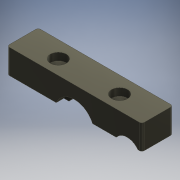
# Autodesk Inventor part: Retainer
Saved by Autodesk Inventor 2016 (Build 200138000, 138)
## iProperties
Created: 2016-11-19
Part Number: Retainer
Material: PC/ABS Plastic
Document SubType Name: Modeling
Designer: Scott
Density: 0.357273 g/cm^3
Appearance: Gunmetal
Author: Scott
## iProperties of the stored document Retainer_3DPrint.ipt
Created: 2017-03-26
Part Number: Retainer_3DPrint
Material: Generic
Document SubType Name: Modeling
Designer: Scott
Density: 1 g/cm^3
Appearance: Default
Author: Scott
Autodesk Inventor part; units mm, degrees
ref_plane "XZ Plane" through (0, 0, 0) normal (0, 1, 0) x (-1, 0, 0)
ref_plane "XY Plane" through (0, 0, 0) normal (0, 0, 1) x (1, 0, 0)
sketch "Sketch1" plane through (0, 0, 0) normal (0, 0, 1) x (1, 0, 0)
  line L0 (-27.5, 6.775) -> (27.5, 6.775)
  line L1 (27.5, 6.775) -> (27.5, -5.925)
  line L2 (27.5, -5.925) -> (-27.5, -5.925)
  line L3 (-27.5, -5.925) -> (-27.5, 6.775)
  point P0 (0, 0)
  dimension "d0" = 6.775
  dimension "d1" = 5.925
  dimension "d2" = 27.5
  dimension "d3" = 27.5
  constraints: 8 end point, 2 parallel, 1 horizontal, 1 perpendicular
  measures "d0" distance from line of point (0, 0) L0
  measures "d1" distance from line of L2 point (0, 0)
  measures "d2" distance from line of L3 point (0, 0)
  measures "d3" distance from line of point (0, 0) L1
extrude "Extrusion1" add sketch "Sketch1" along normal blind 10
ref_plane "Work Plane1" through (0, 0, -3.25) normal (0, 0, -1) x (-1, 0, 0)
sketch "Sketch2" plane through (0, 0, -3.25) normal (0, 0, -1) x (-1, 0, 0)
  line L0 (27.5, 6.775) -> (-27.5, 6.775) projected
  line L1 (-27.5, -5.925) -> (27.5, -5.925) projected
  line L2 (0, 6.775) -> (-8.1, 6.775)
  line L3 (-27.5, 6.775) -> (27.5, 6.775) projected
  line L4 (-8.1, 6.775) -> (-8.1, 2.825)
  line L5 (-8.1, 2.825) -> (-6.25, 2.825)
  line L6 (-6.25, 2.825) -> (-6.25, -2.825)
  line L7 (-6.25, -2.825) -> (-8.1, -2.825)
  line L8 (-8.1, -2.825) -> (-8.1, -5.925)
  line L9 (27.5, -5.925) -> (-27.5, -5.925) projected
  line L10 (-8.1, -5.925) -> (0, -5.925)
  line L11 (0, -5.925) -> (0, 6.775)
  line L12 (0, -8.465) -> (0, 9.315) projected
  point P0 (0, 0)
  dimension "d7" = 8.1
  dimension "d8" = 6.25
  dimension "d9" = 3.95
  dimension "d10" = 3.1
  constraints: 16 end point, 4 perpendicular, 4 point on line, 2 midpoint, 1 vertical
  measures "d7" distance between parallel lines of L11 L4
  measures "d8" distance between parallel lines of L11 L6
  measures "d9" distance of L2.end L4.end
  measures "d10" distance of L7.end L8.end
revolve "Revolution1" cut sketch "Sketch2" angle 180 about axis through (0, 0, -3.25) along (0, -1, 0)
sketch "Sketch3" plane through (0, 0, 10) normal (0, 0, 1) x (1, 0, 0)
  line L0 (0, 0) -> (43.2339, 0) construction
  line L1 (0, 0) -> (-39.8542, 0) construction
  point P0 (-12.5, 0)
  point P1 (12.5, 0)
  dimension "d12" = 12.5
  dimension "d13" = 12.5
  constraints: 4 end point, 2 horizontal, 2 point on line
  measures "d12" distance of L0.start point (-12.5, 0)
  measures "d13" distance of point (12.5, 0) L0.start
hole "Hole1" at (-12.5, 0, 10) at (12.5, 0, 10) direction (0, 0, -1) diameter 3.5 end through all counterbore diameter 6.5 counterbore depth 3
sketch "Sketch5" plane through (-27.5, 6.775, 10) normal (0, 1, 0) x (1, 0, 0)
  arc A0 (22.1615, 10) -> (32.8385, 10) centre (27.5, 13.25) ccw projected
  line L0 (27.5, 13.25) -> (61.0026, 13.25) construction
  line L1 (55, 10) -> (55, 0) projected
  circle A1 centre (49, 13.25) radius 5.5
  point P0 (27.5, 10)
  dimension "d26" = 6
  dimension "d27" = 11
  constraints: 2 end point, 1 centre point, 1 horizontal, 1 point on line
  measures "d26" distance from line of A1.centre L1
  measures "d27" diameter of A1
extrude "Extrusion3" cut sketch "Sketch5" against normal through all
sketch "Sketch6" plane through (-12.5, 0, 7) normal (0, 0, 1) x (1, 0, 0)
  circle A0 centre (0, 0) radius 1.75 projected
  circle A1 centre (25, 0) radius 1.75 projected
  point P0 (12.5, 0)
extrude "Extrusion4" add sketch "Sketch6" against normal blind 0.4
fillet "Fillet2" radius 1 4 edges at (-27.5, 6.775, 5) (-27.5, -5.925, 5) (27.5, 6.775, 5) (27.5, -5.925, 5)
equation "\"d3\" = d2"
equation "\"d13\" = d12"
body "Solid1"
